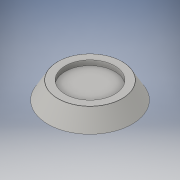
# Autodesk Inventor part: MainBase
Saved by Autodesk Inventor 2016 SP1 (Build 200210100, 210)
## iProperties
Created: 2016-02-19
Part Number: MainBase
Material: Generic
Document SubType Name: Modeling
Designer: Tore Den Store
Density: 1 g/cm^3
Appearance: Default
Author: Tore Den Store
Autodesk Inventor part; units mm, degrees
ref_plane "YZ Plane" through (0, 0, 0) normal (1, 0, 0) x (0, 1, 0)
ref_plane "XZ Plane" through (0, 0, 0) normal (0, 1, 0) x (-1, 0, 0)
ref_plane "XY Plane" through (0, 0, 0) normal (0, 0, 1) x (1, 0, 0)
sketch "Sketch2" plane through (0, 0, 0) normal (0, 1, 0) x (-1, 0, 0)
  line L0 (0, 0) -> (1700, 0)
  line L1 (0, 0) -> (0, 500)
  line L2 (0, 500) -> (1000, 500)
  line L3 (1000, 500) -> (1000, 700)
  line L4 (1000, 700) -> (1300, 700)
  line L5 (1300, 700) -> (1700, 0)
  dimension "d0" = 1700
  dimension "d1" = 500
  dimension "d2" = 1000
  dimension "d3" = 200
  dimension "d4" = 300
  constraints: 12 end point, 2 horizontal, 2 perpendicular, 1 vertical
  measures "d0" distance of L0.start L0.end
  measures "d1" distance of L0.start L1.end
  measures "d2" distance of L1.end L2.end
  measures "d3" distance of L2.end L3.end
  measures "d4" distance of L3.end L4.end
revolve "Revolution1" add sketch "Sketch2" angle 360 about axis through (0, 0, 0) along (0, 0, 1)
fillet "Fillet1" radius 10 1 edges at (1300, 0, 700)
body "Solid1"
